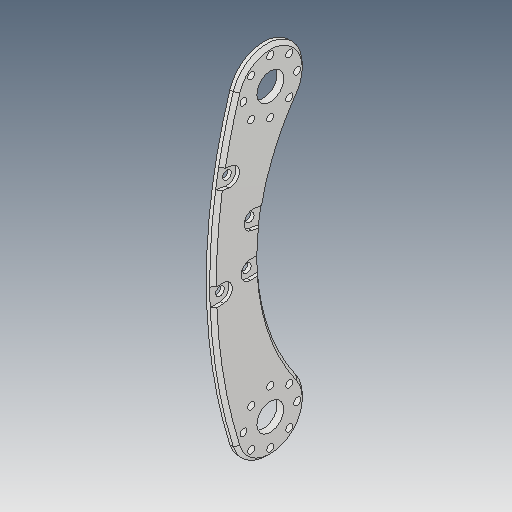
# Autodesk Inventor part: side_frame
Saved by Autodesk Inventor 2019.4 (Build 234330000, 330)
## iProperties
Created: 2018-08-09
Part Number: side_frame
Material: 一般
Document SubType Name: Modeling
Designer: student
Density: 1 g/cm^3
Appearance: 滑らか - 白
Mass: 3.03437 g
Surface Area: 39.651 cm^2
Volume: 3.03437 cm^3
Author: student
Autodesk Inventor part; units mm, degrees
ref_plane "YZ Plane" through (0, 0, 0) normal (1, 0, 0) x (0, 1, 0)
ref_plane "XZ Plane" through (0, 0, 0) normal (0, 1, 0) x (-1, 0, 0)
ref_plane "XY Plane" through (0, 0, 0) normal (0, 0, 1) x (1, 0, 0)
sketch "スケッチ1" plane through (0, 0, 0) normal (1, 0, 0) x (0, 1, 0)
  line L0 (-42.5, 0) -> (42.5, 0) construction
  circle A0 centre (-42.5, 0) radius 4
  circle A1 centre (-42.5, 0) radius 8 construction
  circle A2 centre (-42.5, 8) radius 1.05
  line L1 (-42.5, 8) -> (-42.5, 0) construction
  circle A3 centre (-48.1569, 5.6569) radius 1.05
  circle A4 centre (-50.5, 0) radius 1.05
  circle A5 centre (-48.1569, -5.6569) radius 1.05
  circle A6 centre (-42.5, -8) radius 1.05
  circle A7 centre (-36.8431, -5.6569) radius 1.05
  circle A8 centre (-34.5, 0) radius 1.05
  circle A9 centre (-36.8431, 5.6569) radius 1.05
  arc A10 (-45.6384, 10.02) -> (-36.4408, -8.5753) centre (-42.5, 0) ccw
  arc A11 (36.4408, -8.5753) -> (-36.4408, -8.5753) centre (0, -60.1481) ccw
  arc A12 (45.6384, 10.02) -> (-45.6384, 10.02) centre (0, -135.6923) ccw
  arc A13 (36.4408, -8.5753) -> (45.6384, 10.02) centre (42.5, 0) ccw
  circle A14 centre (42.5, 0) radius 4
  circle A15 centre (42.5, 0) radius 8 construction
  line L2 (42.5, 0) -> (42.5, 8) construction
  circle A16 centre (42.5, 8) radius 1.05
  circle A17 centre (36.8431, 5.6569) radius 1.05
  circle A18 centre (34.5, 0) radius 1.05
  circle A19 centre (36.8431, -5.6569) radius 1.05
  circle A20 centre (42.5, -8) radius 1.05
  circle A21 centre (48.1569, -5.6569) radius 1.05
  circle A22 centre (50.5, 0) radius 1.05
  circle A23 centre (48.1569, 5.6569) radius 1.05
  line L3 (25.1751, 11.8679) -> (10.853, 5.1036) construction
  circle A24 centre (25.1751, 11.8679) radius 1.3
  circle A25 centre (10.853, 5.1036) radius 1.3
  circle A26 centre (25.1751, 11.8679) radius 3 construction
  circle A27 centre (10.853, 5.1036) radius 3 construction
  circle A28 centre (-3.7289, 13.9535) radius 1.3
  circle A29 centre (-1.7302, 5.9774) radius 1.3
  line L4 (0, 3) -> (0, 0) construction
  line L5 (0, 17) -> (0, 3) construction
  line L6 (-3.7289, 13.9535) -> (-1.7302, 5.9774) construction
  circle A30 centre (-3.7289, 13.9535) radius 3 construction
  circle A31 centre (-1.7302, 5.9774) radius 3 construction
  line L7 (-42.5, 0) -> (-2.7295, 9.9655) construction
  line L8 (23.7036, 7.7857) -> (-3.3435, -4.8265) construction
  arc A32 (30.9737, 13.8255) -> (24.6107, -1.9932) centre (42.5, 0) ccw construction
  dimension "d1" = 16
  dimension "d0" = 8
  dimension "d2" = 2.1
  dimension "d5" = 360
  dimension "d7" = 85
  dimension "d8" = 10.5
  dimension "d9" = 2.1
  dimension "d12" = 360
  dimension "d14" = 3
  dimension "d16" = 2.6
  dimension "d17" = 6
  dimension "d30" = 14
  dimension "d35" = 41
  dimension "d36" = 15
  dimension "d39" = 25
  dimension "d40" = 18
  constraints: 31 centre point, 18 end point, 15 point on circle, 14 coincident, 10 tangent, 8 equal radius, 2 midpoint, 2 vertical, 2 vertical alignment, 1 collinear, 1 horizontal, 1 perpendicular, 39 other
  measures "d0" diameter of A0
  measures "d2" diameter of A2
  measures "d7" distance of L0.start L0.end
  measures "d8" radius of A10
  measures "d9" diameter of A16
  measures "d14" distance from line of L0 L4.start
  measures "d16" diameter of A25
  measures "d17" diameter of A27
  measures "d30" distance of L5.start L4.start
  measures "d35" distance of L7.start L7.end
  measures "d36" distance from line of L0.end L8
  measures "d39" angle of L0 L8
  measures "d40" radius of A32
extrude "押し出し1" add sketch "スケッチ1" along normal blind 2
chamfer "面取り1" distance 1 angle 45 4 edges at (2, 0, 17) (2, -51.9117, -4.6552) (2, 0, 3) (2, 51.9117, -4.6552)
sketch "スケッチ2" plane through (2, 0, 0) normal (1, 0, 0) x (0, 0, -1)
  circle A0 centre (-13.9535, -3.7289) radius 1.3 construction
  circle A1 centre (-5.9774, -1.7302) radius 1.3 construction
  arc A2 (8.5753, 36.4408) -> (8.5753, -36.4408) centre (60.1481, 0) ccw construction
  arc A3 (-10.02, 45.6384) -> (-10.02, -45.6384) centre (135.6923, 0) ccw construction
  line L0 (-5.9774, -1.7302) -> (60.1481, 0) construction
  line L1 (-13.9535, -3.7289) -> (135.6923, 0) construction
  line L2 (-13.9535, -3.7289) -> (-16.9526, -3.8036) construction
  arc A4 (-13.8863, -6.428) -> (-14.0208, -1.0297) centre (-13.9535, -3.7289) ccw
  arc A5 (-6.048, 0.9689) -> (-5.9067, -4.4293) centre (-5.9774, -1.7302) ccw
  line L3 (-5.9067, -4.4293) -> (-2.85, -4.3493)
  line L4 (-6.048, 0.9689) -> (-2.9913, 1.0488)
  line L5 (-14.0208, -1.0297) -> (-16.996, -1.1038)
  line L6 (-13.8863, -6.428) -> (-16.8615, -6.5021)
  arc A6 (-16.996, -1.1038) -> (-16.8615, -6.5021) centre (135.6923, 0) ccw
  arc A7 (-2.9913, 1.0488) -> (-2.85, -4.3493) centre (60.1481, 0) ccw
  arc A8 (-12.3219, 22.5135) -> (-11.4138, 27.8366) centre (-11.8679, 25.1751) ccw
  arc A9 (-4.6606, 13.5165) -> (-5.5466, 8.1896) centre (-5.1036, 10.853) ccw
  line L7 (-4.6606, 13.5165) -> (-1.6443, 13.0148)
  line L8 (-5.5466, 8.1896) -> (-2.5303, 7.6879)
  line L9 (-12.3219, 22.5135) -> (-15.2557, 23.014)
  line L10 (-11.4138, 27.8366) -> (-14.3475, 28.3371)
  arc A10 (-14.3475, 28.3371) -> (-15.2557, 23.014) centre (135.6923, 0) ccw
  arc A11 (-1.6443, 13.0148) -> (-2.5303, 7.6879) centre (60.1481, 0) ccw
  circle A12 centre (-5.1036, 10.853) radius 1.3 construction
  circle A13 centre (-11.8679, 25.1751) radius 1.3 construction
  line L11 (-11.8679, 25.1751) -> (135.6923, 0) construction
  line L12 (60.1481, 0) -> (-5.1036, 10.853) construction
  point P0 (0, 0)
  dimension "d25" = 5.4
  constraints: 26 end point, 21 point on circle, 8 centre point, 8 parallel, 8 tangent, 6 concentric, 5 equal radius, 1 collinear
  measures "d25" distance between parallel lines of L5 L6
extrude "押し出し2" cut sketch "スケッチ2" against normal blind 1
